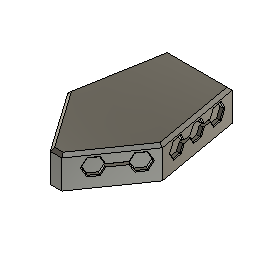
wedge_10deg_34mm (Autodesk Fusion 360 design; units mm, degrees)
Autodesk Fusion 360 part; units mm, degrees
sketch "case_bottom" plane through (0, 0, 0) normal (0, 0, 1) x (1, 0, 0)
  line L0 (-89.5317, -21.1855) -> (-110.379, -22.6565)
  line L1 (-18.858, -113.0832) -> (-40.3079, -82.4999)
  line L2 (-110.379, -22.6565) -> (-131.8327, -31.4447)
  line L3 (-32.6394, -39.0095) -> (-70.5162, -24.5567)
  line L4 (-131.8327, -31.4447) -> (-146.0321, -111.9735)
  line L5 (-70.5162, -24.5567) -> (-70.6053, -24.5227)
  line L6 (-70.6053, -24.5227) -> (-89.5317, -21.1855)
  line L7 (-40.3079, -82.4999) -> (-32.6394, -39.0095)
  line L8 (-146.0321, -111.9735) -> (-30.0269, -132.4284)
  line L9 (-30.0269, -132.4284) -> (-18.858, -113.0832)
  line L10 (-37.1374, -81.7958) -> (-29.2546, -37.09)
  line L11 (-134.5, -29.2953) -> (-149.5075, -114.407)
  line L12 (-111.0705, -19.6978) -> (-134.5, -29.2953)
  line L13 (-28.4791, -135.7475) -> (-15.3035, -112.9267)
  line L14 (-89.3744, -18.1669) -> (-111.0705, -19.6978)
  line L15 (-149.5075, -114.407) -> (-28.4791, -135.7475)
  line L16 (-69.8028, -21.6179) -> (-89.3744, -18.1669)
  line L17 (-29.2546, -37.09) -> (-69.8028, -21.6179)
  line L18 (-15.3035, -112.9267) -> (-37.1374, -81.7958)
  line L19 (-132.8996, -30.5849) -> (-147.4223, -112.9469)
  line L20 (-89.4688, -19.978) -> (-110.6556, -21.473)
  line L21 (-39.0397, -82.2183) -> (-31.2855, -38.2417)
  line L22 (-70.2843, -23.3608) -> (-89.4688, -19.978)
  line L23 (-110.6556, -21.473) -> (-132.8996, -30.5849)
  line L24 (-17.4362, -113.0206) -> (-39.0397, -82.2183)
  line L25 (-31.2855, -38.2417) -> (-70.2843, -23.3608)
  line L26 (-147.4223, -112.9469) -> (-29.4078, -133.756)
  line L27 (-29.4078, -133.756) -> (-17.4362, -113.0206)
  line L28 (-38.4056, -82.0774) -> (-30.6085, -37.8578)
  line L29 (-29.0982, -134.4199) -> (-16.7253, -112.9893)
  line L30 (-148.1173, -113.4336) -> (-29.0982, -134.4199)
  line L31 (-69.8745, -22.8749) -> (-70.1238, -22.7798)
  line L32 (-16.7253, -112.9893) -> (-38.4056, -82.0774)
  line L33 (-110.7939, -20.8813) -> (-133.4331, -30.1551)
  line L34 (-89.4373, -19.3743) -> (-110.7939, -20.8813)
  line L35 (-70.1238, -22.7798) -> (-89.4373, -19.3743)
  line L36 (-133.4331, -30.1551) -> (-148.1173, -113.4336)
  line L37 (-30.6085, -37.8578) -> (-69.8745, -22.8749)
  circle A0 centre (-110.1746, -43.9466) radius 2.2
  circle A1 centre (-116.7732, -81.3693) radius 2.2
  circle A2 centre (-58.9646, -52.9764) radius 2.2
  circle A3 centre (-50.6841, -98.9366) radius 2.2
  line L38 (-111.0238, -114.9885) -> (-107.8981, -97.2619)
  line L39 (-107.8981, -97.2619) -> (-140.3968, -91.5315)
  line L40 (-140.3968, -91.5315) -> (-143.5225, -109.2581)
  line L41 (-143.5225, -109.2581) -> (-111.0238, -114.9885)
  line L42 (-107.0974, -113.0204) -> (-108.1132, -118.7815)
  line L43 (-99.4469, -120.3096) -> (-98.4311, -114.5485)
  line L44 (-98.4311, -114.5485) -> (-107.0974, -113.0204)
  line L45 (-88.377, -120.8755) -> (-87.7692, -117.4287)
  line L46 (-97.2403, -119.3126) -> (-88.377, -120.8755)
  line L47 (-96.6325, -115.8658) -> (-97.2403, -119.3126)
  line L48 (-87.7692, -117.4287) -> (-96.6325, -115.8658)
  line L49 (-35.8089, -106.9233) -> (-28.3546, -101.7038)
  line L50 (-28.3546, -101.7038) -> (-34.6639, -92.6931)
  line L51 (-42.1182, -97.9126) -> (-35.8089, -106.9233)
  line L52 (-34.6639, -92.6931) -> (-42.1182, -97.9126)
  line L53 (-106.0994, -85.3331) -> (-114.5687, -83.8397)
  line L54 (-107.6448, -94.0978) -> (-106.0994, -85.3331)
  line L55 (-116.1142, -92.6045) -> (-107.6448, -94.0978)
  line L56 (-114.5687, -83.8397) -> (-116.1142, -92.6045)
  line L57 (-12.2546, -24.9377) -> (-12.2546, -147.2751) construction
  circle A4 centre (85.6654, -43.9466) radius 2.2
  line L58 (5.5177, -132.4284) -> (-5.6513, -113.0832)
  circle A5 centre (26.1749, -98.9366) radius 2.2
  line L59 (3.8453, -101.7038) -> (10.1547, -92.6931)
  line L60 (122.913, -112.9469) -> (4.8985, -133.756)
  line L61 (45.3653, -22.8749) -> (45.6145, -22.7798)
  line L62 (14.5305, -82.2183) -> (6.7762, -38.2417)
  line L63 (12.6282, -81.7958) -> (4.7454, -37.09)
  line L64 (90.0595, -83.8397) -> (91.605, -92.6045)
  line L65 (46.007, -24.5567) -> (46.096, -24.5227)
  line L66 (45.6145, -22.7798) -> (64.9281, -19.3743)
  line L67 (10.1547, -92.6931) -> (17.609, -97.9126)
  line L68 (4.589, -134.4199) -> (-7.784, -112.9893)
  line L69 (121.5229, -111.9735) -> (5.5177, -132.4284)
  line L70 (13.8964, -82.0774) -> (6.0993, -37.8578)
  line L71 (6.7762, -38.2417) -> (45.775, -23.3608)
  line L72 (124.9982, -114.407) -> (3.9699, -135.7475)
  line L73 (-5.6513, -113.0832) -> (15.7986, -82.4999)
  line L74 (45.2936, -21.6179) -> (64.8652, -18.1669)
  line L75 (17.609, -97.9126) -> (11.2996, -106.9233)
  line L76 (11.2996, -106.9233) -> (3.8453, -101.7038)
  line L77 (6.0993, -37.8578) -> (45.3653, -22.8749)
  line L78 (45.775, -23.3608) -> (64.9595, -19.978)
  line L79 (-7.784, -112.9893) -> (13.8964, -82.0774)
  line L80 (46.096, -24.5227) -> (65.0224, -21.1855)
  line L81 (-7.0731, -113.0206) -> (14.5305, -82.2183)
  line L82 (123.6081, -113.4336) -> (4.589, -134.4199)
  line L83 (15.7986, -82.4999) -> (8.1301, -39.0095)
  line L84 (3.9699, -135.7475) -> (-9.2058, -112.9267)
  line L85 (65.0224, -21.1855) -> (85.8698, -22.6565)
  line L86 (4.7454, -37.09) -> (45.2936, -21.6179)
  line L87 (8.1301, -39.0095) -> (46.007, -24.5567)
  line L88 (-9.2058, -112.9267) -> (12.6282, -81.7958)
  line L89 (4.8985, -133.756) -> (-7.0731, -113.0206)
  circle A6 centre (34.4554, -52.9764) radius 2.2
  line L90 (86.2847, -20.8813) -> (108.9238, -30.1551)
  line L91 (86.5146, -114.9885) -> (83.3889, -97.2619)
  line L92 (73.9218, -114.5485) -> (82.5882, -113.0204)
  line L93 (63.8678, -120.8755) -> (63.26, -117.4287)
  line L94 (63.26, -117.4287) -> (72.1233, -115.8658)
  circle A7 centre (92.264, -81.3693) radius 2.2
  line L95 (81.5901, -85.3331) -> (90.0595, -83.8397)
  line L96 (74.9377, -120.3096) -> (73.9218, -114.5485)
  line L97 (107.3235, -31.4447) -> (121.5229, -111.9735)
  line L98 (115.8875, -91.5315) -> (119.0132, -109.2581)
  line L99 (86.5613, -19.6978) -> (109.9908, -29.2953)
  line L100 (64.9281, -19.3743) -> (86.2847, -20.8813)
  line L101 (64.8652, -18.1669) -> (86.5613, -19.6978)
  line L102 (86.1464, -21.473) -> (108.3904, -30.5849)
  line L103 (109.9908, -29.2953) -> (124.9982, -114.407)
  line L104 (83.3889, -97.2619) -> (115.8875, -91.5315)
  line L105 (119.0132, -109.2581) -> (86.5146, -114.9885)
  line L106 (72.731, -119.3126) -> (63.8678, -120.8755)
  line L107 (72.1233, -115.8658) -> (72.731, -119.3126)
  line L108 (85.8698, -22.6565) -> (107.3235, -31.4447)
  line L109 (108.3904, -30.5849) -> (122.913, -112.9469)
  line L110 (64.9595, -19.978) -> (86.1464, -21.473)
  line L111 (108.9238, -30.1551) -> (123.6081, -113.4336)
  line L112 (82.5882, -113.0204) -> (83.604, -118.7815)
  line L113 (83.1356, -94.0978) -> (81.5901, -85.3331)
  line L114 (91.605, -92.6045) -> (83.1356, -94.0978)
  line L115 (-29.2546, -37.09) -> (4.7454, -37.09)
  line L116 (-15.3035, -112.9267) -> (-9.2058, -112.9267)
  point P0 (-12.2546, -24.9377)
  dimension "d1" = 17
  constraint vertical L57
  constraint coincident L10.end L17.start
  constraint perpendicular L57 L115
  constraint perpendicular L57 L116
  measures "d1" distance of L10.end L57
extrude "Extrude1" add sketch "case_bottom" along normal blind 16.6 contours L10 L18 L63 L88 L115 L116
sketch "Sketch2" plane through (46.9175, -32.906, 0) normal (0.818709, -0.574209, 0) x (0.574209, 0.818709, 0)
  line L0 (-97.7401, 0) -> (-59.7157, 0)
  line L1 (-59.7157, 0) -> (-59.7157, 16.6)
  line L2 (-59.7157, 16.6) -> (-97.7401, 16.6)
  line L3 (-97.7401, 16.6) -> (-97.7401, 0)
  line L4 (-97.7401, 9.7) -> (-59.7157, 9.7) construction
  line L5 (-83.3945, 13.6453) -> (-87.984, 13.704)
  line L6 (-87.984, 13.704) -> (-90.3296, 9.7587)
  line L7 (-90.3296, 9.7587) -> (-88.0857, 5.7547)
  line L8 (-88.0857, 5.7547) -> (-83.4961, 5.696)
  line L9 (-83.4961, 5.696) -> (-81.1505, 9.6413)
  line L10 (-81.1505, 9.6413) -> (-83.3945, 13.6453)
  line L11 (-72.3052, 9.6413) -> (-69.9596, 5.696)
  line L12 (-69.9596, 5.696) -> (-65.3701, 5.7547)
  line L13 (-65.3701, 5.7547) -> (-63.1261, 9.7587)
  line L14 (-63.1261, 9.7587) -> (-65.4717, 13.704)
  line L15 (-65.4717, 13.704) -> (-70.0613, 13.6453)
  line L16 (-70.0613, 13.6453) -> (-72.3052, 9.6413)
  line L17 (-85.7401, 8.95) -> (-67.7157, 8.95)
  arc A0 (-67.7157, 8.95) -> (-67.7157, 10.45) centre (-67.7157, 9.7) ccw
  line L18 (-67.7157, 10.45) -> (-85.7401, 10.45)
  arc A1 (-85.7401, 10.45) -> (-85.7401, 8.95) centre (-85.7401, 9.7) ccw
  line L19 (-85.7401, 9.7) -> (-67.7157, 9.7) construction
  point P0 (-85.7401, 9.7)
  point P1 (-67.7157, 9.7)
  point P2 (-85.7401, 9.7)
  point P3 (-67.7157, 9.7)
  dimension "d4" = 6.9
  dimension "d5" = 8
  dimension "d6" = 12
  dimension "d7" = 3.975
  dimension "d8" = 3.975
  dimension "d9" = 1.5
  constraint coincident L3 L4.start
  constraint coincident L1 L4.end
  constraint perpendicular L1 L4
  constraint coincident L4 P2
  constraint coincident L4 P3
  constraint coincident P2 P0
  constraint coincident P3 P1
  constraint tangent L17 A0
  constraint tangent A0 L18
  constraint parallel L17 L18
  constraint tangent L18 A1
  constraint tangent L17 A1
  constraint parallel L4 L19
  measures "d4" distance of L2 L4
  measures "d5" distance of L1 P3
  measures "d6" distance of L3 P2
  measures "d7" distance of P2 L10
  measures "d8" distance of P3 L16
  measures "d9" diameter of A0
sketch "Sketch3" plane through (-1.7405, -0.3069, 0) normal (0.984808, 0.173648, 0) x (-0.173648, 0.984808, 0)
  line L0 (-82.746, 0) -> (-37.3506, 0)
  line L1 (-37.3506, 0) -> (-37.3506, 16.6)
  line L2 (-37.3506, 16.6) -> (-82.746, 16.6)
  line L3 (-82.746, 16.6) -> (-82.746, 0)
  line L4 (-82.746, 9.7) -> (-37.3506, 9.7) construction
  line L5 (-70.7716, 13.6855) -> (-75.3615, 13.6644)
  line L6 (-75.3615, 13.6644) -> (-77.6382, 9.6789)
  line L7 (-77.6382, 9.6789) -> (-75.3249, 5.7145)
  line L8 (-75.3249, 5.7145) -> (-70.735, 5.7356)
  line L9 (-70.735, 5.7356) -> (-68.4584, 9.7211)
  line L10 (-68.4584, 9.7211) -> (-70.7716, 13.6855)
  line L11 (-57.7716, 13.6855) -> (-62.3615, 13.6644)
  line L12 (-62.3615, 13.6644) -> (-64.6382, 9.6789)
  line L13 (-64.6382, 9.6789) -> (-62.3249, 5.7145)
  line L14 (-62.3249, 5.7145) -> (-57.735, 5.7356)
  line L15 (-57.735, 5.7356) -> (-55.4584, 9.7211)
  line L16 (-55.4584, 9.7211) -> (-57.7716, 13.6855)
  line L17 (-44.7716, 13.6855) -> (-49.3615, 13.6644)
  line L18 (-49.3615, 13.6644) -> (-51.6382, 9.6789)
  line L19 (-51.6382, 9.6789) -> (-49.3249, 5.7145)
  line L20 (-49.3249, 5.7145) -> (-44.735, 5.7356)
  line L21 (-44.735, 5.7356) -> (-42.4584, 9.7211)
  line L22 (-42.4584, 9.7211) -> (-44.7716, 13.6855)
  line L23 (-73.0483, 8.95) -> (-47.0483, 8.95)
  arc A0 (-47.0483, 8.95) -> (-47.0483, 10.45) centre (-47.0483, 9.7) ccw
  line L24 (-47.0483, 10.45) -> (-73.0483, 10.45)
  arc A1 (-73.0483, 10.45) -> (-73.0483, 8.95) centre (-73.0483, 9.7) ccw
  line L25 (-73.0483, 9.7) -> (-47.0483, 9.7) construction
  point P0 (-60.0483, 9.7)
  point P1 (-47.0483, 9.7)
  point P2 (-73.0483, 9.7)
  point P3 (-73.0483, 9.7)
  point P4 (-60.0483, 9.7)
  point P5 (-47.0483, 9.7)
  dimension "d10" = 6.9
  dimension "d11" = 13
  dimension "d12" = 13
  dimension "d13" = 3.975
  dimension "d14" = 3.975
  dimension "d15" = 3.975
  dimension "d16" = 1.5
  constraint coincident L3 L4.start
  constraint coincident L1 L4.end
  constraint perpendicular L1 L4
  constraint midpoint L4 P4
  constraint coincident L4 P5
  constraint coincident L4 P3
  constraint coincident P3 P2
  constraint coincident P4 P0
  constraint coincident P5 P1
  constraint tangent L23 A0
  constraint tangent A0 L24
  constraint parallel L23 L24
  constraint tangent L24 A1
  constraint tangent L23 A1
  constraint parallel L4 L25
  measures "d10" distance of L2 L4
  measures "d11" distance of P4 P3
  measures "d12" distance of P4 P5
  measures "d13" distance of P3 L10
  measures "d14" distance of P4 L16
  measures "d15" distance of P5 L22
  measures "d16" diameter of A0
extrude "Extrude2" cut sketch "Sketch3" against normal blind 2 contours L5 L6 L7 L8 L9 L10 L23 L24 A1 | L9 L10 L12 L13 L23 L24 | L9 L10 L23 L24 A1 | L12 L13 L15 L16 L23 L24 | L11 L12 L16 L24 | L15 L16 L18 L19 L23 L24 | L13 L14 L15 L23 | L18 L19 L23 A0 L24 | L17 L18 L19 L20 L21 L22 L23 A0 L24
extrude "Extrude3" cut sketch "Sketch2" against normal blind 2 contours L5 L6 L7 L8 L9 L10 L17 L18 A1 | L9 L10 L11 L16 L17 L18 | L9 L10 L17 L18 A1 | L11 L16 L17 A0 L18 | L11 L12 L13 L14 L15 L16 L17 A0 L18
sketch "Sketch4" plane through (-63.3456, -44.4281, 0) normal (-0.818709, -0.574209, 0) x (0.574209, -0.818709, 0)
  line L0 (45.6422, 0) -> (83.6666, 0)
  line L1 (83.6666, 0) -> (83.6666, 16.6)
  line L2 (83.6666, 16.6) -> (45.6422, 16.6)
  line L3 (45.6422, 16.6) -> (45.6422, 0)
  line L4 (45.6422, 9.7) -> (83.6666, 9.7) construction
  line L5 (55.9836, 13.6478) -> (51.394, 13.7016)
  line L6 (51.394, 13.7016) -> (49.0526, 9.7538)
  line L7 (49.0526, 9.7538) -> (51.3009, 5.7522)
  line L8 (51.3009, 5.7522) -> (55.8905, 5.6984)
  line L9 (55.8905, 5.6984) -> (58.2318, 9.6462)
  line L10 (58.2318, 9.6462) -> (55.9836, 13.6478)
  line L11 (67.077, 9.6462) -> (69.4184, 5.6984)
  line L12 (69.4184, 5.6984) -> (74.008, 5.7522)
  line L13 (74.008, 5.7522) -> (76.2562, 9.7538)
  line L14 (76.2562, 9.7538) -> (73.9149, 13.7016)
  line L15 (73.9149, 13.7016) -> (69.3253, 13.6478)
  line L16 (69.3253, 13.6478) -> (67.077, 9.6462)
  line L17 (53.6422, 8.95) -> (71.6666, 8.95)
  arc A0 (71.6666, 8.95) -> (71.6666, 10.45) centre (71.6666, 9.7) ccw
  line L18 (71.6666, 10.45) -> (53.6422, 10.45)
  arc A1 (53.6422, 10.45) -> (53.6422, 8.95) centre (53.6422, 9.7) ccw
  line L19 (53.6422, 9.7) -> (71.6666, 9.7) construction
  point P0 (53.6422, 9.7)
  point P1 (71.6666, 9.7)
  point P2 (53.6422, 9.7)
  point P3 (71.6666, 9.7)
  dimension "d21" = 6.9
  dimension "d22" = 8
  dimension "d23" = 12
  dimension "d24" = 3.975
  dimension "d25" = 3.975
  dimension "d26" = 1.5
  constraint coincident L3 L4.start
  constraint coincident L1 L4.end
  constraint perpendicular L1 L4
  constraint coincident L4 P2
  constraint coincident L4 P3
  constraint coincident P2 P0
  constraint coincident P3 P1
  constraint tangent L17 A0
  constraint tangent A0 L18
  constraint parallel L17 L18
  constraint tangent L18 A1
  constraint tangent L17 A1
  constraint parallel L4 L19
  measures "d21" distance of L2 L4
  measures "d22" distance of L3 P2
  measures "d23" distance of L1 P3
  measures "d24" distance of P2 L10
  measures "d25" distance of P3 L16
  measures "d26" diameter of A0
extrude "Extrude4" cut sketch "Sketch4" against normal blind 2 contours L5 L6 L7 L8 L9 L10 L17 L18 A1 | L9 L10 L11 L16 L17 L18 | L9 L10 L17 L18 A1 | L11 L16 L17 A0 L18 | L11 L12 L13 L14 L15 L16 L17 A0 L18
sketch "Sketch5" plane through (-22.0297, 3.8844, 0) normal (-0.984808, 0.173648, 0) x (-0.173648, -0.984808, 0)
  line L0 (41.6066, 0) -> (87.002, 0)
  line L1 (87.002, 0) -> (87.002, 16.6)
  line L2 (87.002, 16.6) -> (41.6066, 16.6)
  line L3 (41.6066, 16.6) -> (41.6066, 0)
  line L4 (41.6066, 9.7) -> (87.002, 9.7) construction
  line L5 (53.6183, 13.6639) -> (49.0284, 13.686)
  line L6 (49.0284, 13.686) -> (46.7144, 9.722)
  line L7 (46.7144, 9.722) -> (48.9902, 5.7361)
  line L8 (48.9902, 5.7361) -> (53.5801, 5.714)
  line L9 (53.5801, 5.714) -> (55.8941, 9.678)
  line L10 (55.8941, 9.678) -> (53.6183, 13.6639)
  line L11 (66.6183, 13.6639) -> (62.0284, 13.686)
  line L12 (62.0284, 13.686) -> (59.7144, 9.722)
  line L13 (59.7144, 9.722) -> (61.9902, 5.7361)
  line L14 (61.9902, 5.7361) -> (66.5801, 5.714)
  line L15 (66.5801, 5.714) -> (68.8941, 9.678)
  line L16 (68.8941, 9.678) -> (66.6183, 13.6639)
  line L17 (79.6183, 13.6639) -> (75.0284, 13.686)
  line L18 (75.0284, 13.686) -> (72.7144, 9.722)
  line L19 (72.7144, 9.722) -> (74.9902, 5.7361)
  line L20 (74.9902, 5.7361) -> (79.5801, 5.714)
  line L21 (79.5801, 5.714) -> (81.8941, 9.678)
  line L22 (81.8941, 9.678) -> (79.6183, 13.6639)
  line L23 (51.3043, 8.95) -> (77.3043, 8.95)
  arc A0 (77.3043, 8.95) -> (77.3043, 10.45) centre (77.3043, 9.7) ccw
  line L24 (77.3043, 10.45) -> (51.3043, 10.45)
  arc A1 (51.3043, 10.45) -> (51.3043, 8.95) centre (51.3043, 9.7) ccw
  line L25 (51.3043, 9.7) -> (77.3043, 9.7) construction
  point P0 (51.3043, 9.7)
  point P1 (64.3043, 9.7)
  point P2 (77.3043, 9.7)
  point P3 (51.3043, 9.7)
  point P4 (64.3043, 9.7)
  point P5 (77.3043, 9.7)
  dimension "d29" = 6.9
  dimension "d30" = 13
  dimension "d31" = 13
  dimension "d32" = 3.975
  dimension "d33" = 3.975
  dimension "d34" = 3.975
  dimension "d35" = 1.5
  constraint coincident L3 L4.start
  constraint coincident L1 L4.end
  constraint perpendicular L1 L4
  constraint coincident L4 P3
  constraint midpoint L4 P4
  constraint coincident L4 P5
  constraint coincident P3 P0
  constraint coincident P4 P1
  constraint coincident P5 P2
  constraint tangent L23 A0
  constraint tangent A0 L24
  constraint parallel L23 L24
  constraint tangent L24 A1
  constraint tangent L23 A1
  constraint parallel L4 L25
  measures "d29" distance of L2 L4
  measures "d30" distance of P3 P4
  measures "d31" distance of P4 P5
  measures "d32" distance of P3 L10
  measures "d33" distance of P4 L16
  measures "d34" distance of P5 L22
  measures "d35" diameter of A0
extrude "Extrude5" cut sketch "Sketch5" against normal blind 2 contours L5 L6 L7 L8 L9 L10 L23 L24 A1 | L9 L10 L12 L13 L23 L24 | L9 L10 L23 L24 A1 | L12 L13 L15 L16 L23 L24 | L11 L12 L16 L24 | L15 L16 L18 L19 L23 L24 | L13 L14 L15 L23 | L18 L19 L23 A0 L24 | L17 L18 L19 L20 L21 L22 L23 A0 L24
chamfer "Chamfer1" distance 0.4 angle 45 60 edges at (-4.2772, -105.8995, 11.7313) (-2.2861, -103.0606, 13.6747) (-4.3064, -105.9411, 7.7567) (-2.3444, -103.1438, 5.7253) (-0.4713, -100.4731, 7.323) (-0.4542, -100.4487, 12.0477) (6.1735, -90.9988, 12.0477) (8.0054, -88.387, 13.6747) (6.1906, -90.9745, 7.323) (8.0637, -88.3038, 5.7253) (10.0256, -85.5065, 7.7567) (9.9965, -85.5481, 11.7313) (11.5436, -75.6445, 11.6716) (11.5404, -75.6265, 7.6967) (10.9474, -72.2634, 13.675) (10.941, -72.2274, 5.725) (10.3831, -69.0632, 7.3428) (10.385, -69.0737, 12.0678) (9.2479, -62.6251, 12.0572) (8.69, -59.4609, 13.675) (9.246, -62.6146, 7.3322) (8.6836, -59.4249, 5.725) (8.1257, -56.2607, 7.3428) (8.1275, -56.2712, 12.0678) (6.9905, -49.8226, 12.0572) (6.4325, -46.6584, 13.675) (5.8332, -43.2593, 11.7033) (5.83, -43.2413, 7.7284) (6.4262, -46.6224, 5.725) (6.9886, -49.8121, 7.3322) (-30.3425, -43.2597, 11.704) (-30.3392, -43.2409, 7.729) (-30.9353, -46.6216, 5.725) (-31.4978, -49.8119, 7.332) (-30.9419, -46.6592, 13.675) (-31.4998, -49.8228, 12.057) (-32.6368, -56.2714, 12.068) (-33.1993, -59.4617, 13.675) (-32.6349, -56.2604, 7.343) (-33.1927, -59.4241, 5.725) (-33.7553, -62.6144, 7.332) (-33.7572, -62.6253, 12.057) (-34.8942, -69.0739, 12.068) (-35.4568, -72.2642, 13.675) (-34.8923, -69.0629, 7.343) (-35.4502, -72.2266, 5.725) (-36.0496, -75.6261, 7.696) (-36.0529, -75.6449, 11.671) (-34.507, -85.5463, 11.7277) (-34.5337, -85.5082, 7.753) (-32.5705, -88.3073, 5.7253) (-30.6991, -90.9755, 7.3242) (-32.517, -88.3835, 13.6747) (-30.6835, -90.9978, 12.0489) (-24.0543, -100.4498, 12.0489) (-22.2207, -103.064, 13.6747) (-20.2308, -105.9013, 11.7277) (-20.2041, -105.9394, 7.753) (-22.1673, -103.1403, 5.7253) (-24.0386, -100.4721, 7.3242)
chamfer "Chamfer2" distance 1.5 angle 45 1 faces at (-6.588, -66.8939, 16.6)
